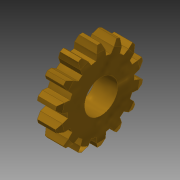
# Autodesk Inventor part: Zahnrad Messing z14
Saved by Autodesk Inventor 2019.3 (Build 233278000, 278)
## iProperties
Category: PARTsolutions
Company: MAEDLER
Created: 2018-08-20
Part Number: Zahnrad Messing z14
Material: Messing, weicher Gelbton, geschweißt
Catalog Web Link: www.cadenas.de
Description: Stzr Messing Ms58-Spur Gears, Brass, Helical Tooth Right Hand, with one-sided hub
Vendor: MAEDLER
Document SubType Name: Modeling
Designer: psadmin
Manufacturer: MAEDLER
Mass: 1.1 g
Surface Area: 2.48322 cm^2
Volume: 0.134968 cm^3
Density: 8.15007 g/cm^3
Appearance: Schweißnaht - Messing
PSOL_IDENT_0: {$CADENAS_DATA\23d-libs\maedler\antriebselemente\stirnzahnraeder\stirnzahnraeder_messing\stzr_messin
PSOL_IDENT_1: g_ms58.prj},204 {VTYP=3D},{NB=Stzr Messing Ms58 26101400},{LINA=Stzr Messing Ms58 26101400},{NN=Stzr
PSOL_IDENT_2: Messing Ms58},{DATE=03.08.2018 09:08:56},{GEOMDATE=26.07.2018 09:15:44},{VERSION=},{LINEID=210},{WB
PSOL_IDENT_3: VAR=},{WBNUMERIC=}  {NB=Stzr Messing Ms58 26101400},{LINA=Stzr Messing Ms58 26101400},{KT=DUMMY},{AR
PSOL_IDENT_4: TNR=26101400},{WST=Messing (Ms58)},{M=0.5},{Z=14},{PDF=PDF Katalogseite},{B1=2.0},{DA=8.00},{D=7.00}
PSOL_IDENT_5: ,{NL=4},{ND=5},{B=2.00},{MD=0.7},{GEW=1.100}
NN: Stzr Messing Ms58
NT: Spur Gears, Brass, Helical Tooth Right Hand, with one-sided hub
NB: Stzr Messing Ms58 26101400
NBSYN: Stzr Messing Ms58 $ARTNR.
LINA: Stzr Messing Ms58 26101400
ARTNR: 26101400
WST: Messing (Ms58)
M: 0.5
Z: 14
PDF: PDF Katalogseite
B1: 2
DA: 8
D: 7
NL: 4
ND: 5
B: 2
MD: 0.7
GEW: 1.1
SUPPLIER: MAEDLER
ARTICLENO: Stzr Messing Ms58 26101400
BOMINFO: Stzr Messing Ms58 26101400
CREATOR: CADENAS GmbH
Title: Stzr Messing Ms58 26101400
Author: Cadenas PARTsolutions
Comments: Spur Gears, Brass, Helical Tooth Right Hand, with one-sided hub
Autodesk Inventor part; units mm, degrees
ref_plane "YZ Plane" through (0, 0, 0) normal (1, 0, 0) x (0, 1, 0)
ref_plane "XZ Plane" through (0, 0, 0) normal (0, 1, 0) x (-1, 0, 0)
ref_plane "XY Plane" through (0, 0, 0) normal (0, 0, 1) x (1, 0, 0)
sketch "Skizze_1" plane through (0, 0, 0) normal (0, 0, 1) x (1, 0, 0)
  line L0 (6, 0) -> (0, 0)
  line L1 (0, 1) -> (6, 1)
  line L2 (6, 1) -> (6, 2.5)
  line L3 (6, 2.5) -> (2, 2.5)
  line L4 (2, 2.5) -> (2, 3.5)
  line L5 (2, 3.5) -> (1, 6.2475)
  line L6 (1, 6.2475) -> (0, 3.5)
  line L7 (0, 3.5) -> (0, 1)
  constraints: 16 end point
revolve "Revolution1" add sketch "Skizze_1" angle 360 about axis through (6, 0, 0) along (1, 0, 0)
sketch "Skizze_2" plane through (2, 0, 0) normal (1, 0, 0) x (0, 0, -1)
  circle A0 centre (0, 0) radius 12
  arc A1 (-3.9965, 0.1667) -> (-3.9965, -0.1667) centre (0, 0) ccw
  line L0 (-3.9965, -0.1667) -> (-3.479, -0.3829)
  line L1 (-3.479, -0.3829) -> (-2.9665, -0.4471)
  arc A2 (-2.9665, -0.4471) -> (-2.8667, -0.8843) centre (0, 0) ccw
  line L2 (-2.8667, -0.8843) -> (-3.3006, -1.1645)
  line L3 (-3.3006, -1.1645) -> (-3.6731, -1.5839)
  arc A3 (-3.6731, -1.5839) -> (-3.5284, -1.8842) centre (0, 0) ccw
  line L4 (-3.5284, -1.8842) -> (-2.9683, -1.8545)
  line L5 (-2.9683, -1.8545) -> (-2.4787, -1.69)
  arc A4 (-2.4787, -1.69) -> (-2.1992, -2.0405) centre (0, 0) ccw
  line L6 (-2.1992, -2.0405) -> (-2.4685, -2.4812)
  line L7 (-2.4685, -2.4812) -> (-2.6221, -3.0207)
  arc A5 (-2.6221, -3.0207) -> (-2.3615, -3.2285) centre (0, 0) ccw
  line L8 (-2.3615, -3.2285) -> (-1.8698, -2.9587)
  line L9 (-1.8698, -2.9587) -> (-1.5, -2.5981)
  arc A6 (-1.5, -2.5981) -> (-1.096, -2.7926) centre (0, 0) ccw
  line L10 (-1.096, -2.7926) -> (-1.1475, -3.3066)
  line L11 (-1.1475, -3.3066) -> (-1.0518, -3.8592)
  arc A7 (-1.0518, -3.8592) -> (-0.7268, -3.9334) centre (0, 0) ccw
  line L12 (-0.7268, -3.9334) -> (-0.4008, -3.477)
  line L13 (-0.4008, -3.477) -> (-0.2242, -2.9916)
  arc A8 (-0.2242, -2.9916) -> (0.2242, -2.9916) centre (0, 0) ccw
  line L14 (0.2242, -2.9916) -> (0.4008, -3.477)
  line L15 (0.4008, -3.477) -> (0.7268, -3.9334)
  arc A9 (0.7268, -3.9334) -> (1.0518, -3.8592) centre (0, 0) ccw
  line L16 (1.0518, -3.8592) -> (1.1475, -3.3066)
  line L17 (1.1475, -3.3066) -> (1.096, -2.7926)
  arc A10 (1.096, -2.7926) -> (1.5, -2.5981) centre (0, 0) ccw
  line L18 (1.5, -2.5981) -> (1.8698, -2.9587)
  line L19 (1.8698, -2.9587) -> (2.3615, -3.2285)
  arc A11 (2.3615, -3.2285) -> (2.6221, -3.0207) centre (0, 0) ccw
  line L20 (2.6221, -3.0207) -> (2.4685, -2.4812)
  line L21 (2.4685, -2.4812) -> (2.1992, -2.0405)
  arc A12 (2.1992, -2.0405) -> (2.4787, -1.69) centre (0, 0) ccw
  line L22 (2.4787, -1.69) -> (2.9683, -1.8545)
  line L23 (2.9683, -1.8545) -> (3.5284, -1.8842)
  arc A13 (3.5284, -1.8842) -> (3.6731, -1.5839) centre (0, 0) ccw
  line L24 (3.6731, -1.5839) -> (3.3006, -1.1645)
  line L25 (3.3006, -1.1645) -> (2.8667, -0.8843)
  arc A14 (2.8667, -0.8843) -> (2.9665, -0.4471) centre (0, 0) ccw
  line L26 (2.9665, -0.4471) -> (3.479, -0.3829)
  line L27 (3.479, -0.3829) -> (3.9965, -0.1667)
  arc A15 (3.9965, -0.1667) -> (3.9965, 0.1667) centre (0, 0) ccw
  line L28 (3.9965, 0.1667) -> (3.479, 0.3829)
  line L29 (3.479, 0.3829) -> (2.9665, 0.4471)
  arc A16 (2.9665, 0.4471) -> (2.8667, 0.8843) centre (0, 0) ccw
  line L30 (2.8667, 0.8843) -> (3.3006, 1.1645)
  line L31 (3.3006, 1.1645) -> (3.6731, 1.5839)
  arc A17 (3.6731, 1.5839) -> (3.5284, 1.8842) centre (0, 0) ccw
  line L32 (3.5284, 1.8842) -> (2.9683, 1.8545)
  line L33 (2.9683, 1.8545) -> (2.4787, 1.69)
  arc A18 (2.4787, 1.69) -> (2.1992, 2.0405) centre (0, 0) ccw
  line L34 (2.1992, 2.0405) -> (2.4685, 2.4812)
  line L35 (2.4685, 2.4812) -> (2.6221, 3.0207)
  arc A19 (2.6221, 3.0207) -> (2.3615, 3.2285) centre (0, 0) ccw
  line L36 (2.3615, 3.2285) -> (1.8698, 2.9587)
  line L37 (1.8698, 2.9587) -> (1.5, 2.5981)
  arc A20 (1.5, 2.5981) -> (1.096, 2.7926) centre (0, 0) ccw
  line L38 (1.096, 2.7926) -> (1.1475, 3.3066)
  line L39 (1.1475, 3.3066) -> (1.0518, 3.8592)
  arc A21 (1.0518, 3.8592) -> (0.7268, 3.9334) centre (0, 0) ccw
  line L40 (0.7268, 3.9334) -> (0.4008, 3.477)
  line L41 (0.4008, 3.477) -> (0.2242, 2.9916)
  arc A22 (0.2242, 2.9916) -> (-0.2242, 2.9916) centre (0, 0) ccw
  line L42 (-0.2242, 2.9916) -> (-0.4008, 3.477)
  line L43 (-0.4008, 3.477) -> (-0.7268, 3.9334)
  arc A23 (-0.7268, 3.9334) -> (-1.0518, 3.8592) centre (0, 0) ccw
  line L44 (-1.0518, 3.8592) -> (-1.1475, 3.3066)
  line L45 (-1.1475, 3.3066) -> (-1.096, 2.7926)
  arc A24 (-1.096, 2.7926) -> (-1.5, 2.5981) centre (0, 0) ccw
  line L46 (-1.5, 2.5981) -> (-1.8698, 2.9587)
  line L47 (-1.8698, 2.9587) -> (-2.3615, 3.2285)
  arc A25 (-2.3615, 3.2285) -> (-2.6221, 3.0207) centre (0, 0) ccw
  line L48 (-2.6221, 3.0207) -> (-2.4685, 2.4812)
  line L49 (-2.4685, 2.4812) -> (-2.1992, 2.0405)
  arc A26 (-2.1992, 2.0405) -> (-2.4787, 1.69) centre (0, 0) ccw
  line L50 (-2.4787, 1.69) -> (-2.9683, 1.8545)
  line L51 (-2.9683, 1.8545) -> (-3.5284, 1.8842)
  arc A27 (-3.5284, 1.8842) -> (-3.6731, 1.5839) centre (0, 0) ccw
  line L52 (-3.6731, 1.5839) -> (-3.3006, 1.1645)
  line L53 (-3.3006, 1.1645) -> (-2.8667, 0.8843)
  arc A28 (-2.8667, 0.8843) -> (-2.9665, 0.4471) centre (0, 0) ccw
  line L54 (-2.9665, 0.4471) -> (-3.479, 0.3829)
  line L55 (-3.479, 0.3829) -> (-3.9965, 0.1667)
  constraints: 112 end point, 56 point on circle, 29 centre point
extrude "Extrusion1" cut sketch "Skizze_2" along normal mid plane 12
sketch "Skizze3" plane through (6, 0, 0) normal (1, 0, 0) x (0, 0, -1)
  circle A0 centre (0, 0) radius 2.5 projected
extrude "Extrusion2" cut sketch "Skizze3" against normal blind 4
sketch "Skizze4" plane through (0, 0, 0) normal (-1, 0, 0) x (0, 0, 1)
  point P0 (0, 0)
  point P1 (0, 0)
  constraints: 1 coincident
hole "Bohrung1" at (0, 0, 0) direction (1, 0, 0) diameter 3 end through all
body "Solid1"
